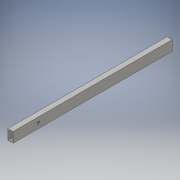
# Autodesk Inventor part: ArmBar
Saved by Autodesk Inventor 2016 (Build 200138000, 138)
## iProperties
Created: 2016-01-25
Part Number: ArmBar
Material: Generic
Document SubType Name: Modeling
Designer: Mentor1102
Density: 1 g/cm^3
Appearance: Default
Author: Mentor1102
Autodesk Inventor part; units mm, degrees
ref_plane "YZ Plane" through (0, 0, 0) normal (1, 0, 0) x (0, 1, 0)
ref_plane "XZ Plane" through (0, 0, 0) normal (0, 1, 0) x (-1, 0, 0)
ref_plane "XY Plane" through (0, 0, 0) normal (0, 0, 1) x (1, 0, 0)
sketch "Sketch1" plane through (0, 0, 0) normal (0, 0, 1) x (1, 0, 0)
  line L0 (0, 25.4) -> (25.4, 25.4)
  line L1 (25.4, 25.4) -> (25.4, 76.2)
  line L2 (25.4, 76.2) -> (0, 76.2)
  line L3 (0, 76.2) -> (0, 25.4)
  line L4 (0, 25.4) -> (3.175, 25.4)
  line L5 (3.175, 25.4) -> (3.175, 28.575) construction
  line L6 (25.4, 76.2) -> (22.225, 76.2)
  line L7 (22.225, 76.2) -> (22.225, 73.025) construction
  line L8 (3.175, 28.575) -> (22.225, 28.575)
  line L9 (22.225, 28.575) -> (22.225, 73.025)
  line L10 (22.225, 73.025) -> (3.175, 73.025)
  line L11 (3.175, 73.025) -> (3.175, 28.575)
  point P0 (0, 0)
  dimension "d0" = 25.4
  dimension "d1" = 50.8
  dimension "d2" = 3.175
  dimension "d3" = 3.175
  dimension "d4" = 3.175
  dimension "d5" = 3.175
  constraints: 24 end point, 5 parallel, 3 perpendicular, 2 horizontal, 2 point on line
  measures "d0" distance of L2.end L1.end
  measures "d1" distance of L1.end L0.end
  measures "d2" distance of L0.start L4.end
  measures "d3" distance of L4.end L5.end
  measures "d4" distance of L1.end L6.end
  measures "d5" distance of L6.end L7.end
extrude "Extrusion1" add sketch "Sketch1" along normal blind 765.175
sketch "Sketch3" plane through (25.4, 25.4, 0) normal (1, 0, 0) x (0, 0, -1)
  line L0 (0, 0) -> (0, 50.8) projected
  line L1 (0, 50.8) -> (-765.175, 50.8) projected
  line L2 (-765.175, 0) -> (-765.175, 50.8) projected
  line L3 (0, 0) -> (-765.175, 0) projected
  line L4 (-765.175, 50.8) -> (-765.175, 0) projected
  line L5 (-765.175, 25.4) -> (-638.175, 25.4) construction
  circle A0 centre (-638.175, 25.4) radius 6.35
  point P0 (0, -25.4)
  dimension "d13" = 127
  dimension "d14" = 12.7
  constraints: 2 end point, 1 centre point, 1 coincident, 1 horizontal, 1 midpoint
  measures "d13" distance of L5.start L5.end
  measures "d14" diameter of A0
extrude "Extrusion3" cut sketch "Sketch3" against normal through all contours A0
sketch "Sketch4" plane through (0, 0, 0) normal (0, 0, -1) x (-1, 0, 0)
  line L0 (-3.175, 73.025) -> (-3.175, 28.575) projected
  line L1 (-3.175, 28.575) -> (-22.225, 28.575) projected
  line L2 (-22.225, 28.575) -> (-22.225, 73.025) projected
  line L3 (-22.225, 73.025) -> (-3.175, 73.025) projected
  line L4 (0, 25.4) -> (-25.4, 25.4) projected
  line L5 (0, 76.2) -> (0, 25.4) projected
  line L6 (-25.4, 76.2) -> (0, 76.2) projected
  line L7 (-25.4, 25.4) -> (-25.4, 76.2) projected
  point P0 (0, 0)
extrude "Extrusion4" add sketch "Sketch4" along normal blind 25.4
body "Solid1"
